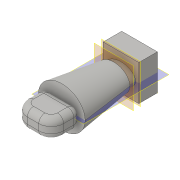
# Autodesk Inventor part: maleNT2
Saved by Autodesk Inventor 2016 (Build 200138000, 138)
## iProperties
Created: 2016-01-27
Part Number: maleNT2
Material: Generic
Document SubType Name: Modeling
Designer: 301278
Density: 1 g/cm^3
Appearance: Default
Author: 301278
Autodesk Inventor part; units mm, degrees
ref_plane "YZ Plane" through (0, 0, 0) normal (1, 0, 0) x (0, 1, 0)
ref_plane "XZ Plane" through (0, 0, 0) normal (0, 1, 0) x (-1, 0, 0)
ref_plane "XY Plane" through (0, 0, 0) normal (0, 0, 1) x (1, 0, 0)
sketch "Sketch1" plane through (0, 0, 0) normal (0, 0, 1) x (1, 0, 0)
  line L0 (0, 0) -> (14.605, 0)
  line L1 (14.605, 0) -> (14.605, 14.605)
  line L2 (14.605, 14.605) -> (0, 14.605)
  line L3 (0, 14.605) -> (0, 0)
  dimension "d0" = 14.605
  dimension "d1" = 14.605
  constraints: 8 end point, 2 parallel, 1 horizontal, 1 perpendicular
  measures "d0" distance of L2.end L1.end
  measures "d1" distance of L1.end L0.end
extrude "Extrusion1" add sketch "Sketch1" along normal blind 7.62
ref_plane "Work Plane1" through (0, 14.605, 7.62) normal (0, 0, 1) x (1, 0, 0)
sketch "Sketch2" plane through (0, 14.605, 7.62) normal (0, 0, 1) x (1, 0, 0)
  line L0 (14.605, 0) -> (0, 0) construction
  line L1 (0, 0) -> (7.3025, 0) construction
  line L2 (7.3025, 0) -> (14.605, 0) construction
  line L3 (7.3025, 0) -> (7.3025, -7.3025) construction
  ellipse E0 centre (7.3025, -7.3025) end of major axis (13.2969, -7.3025) minor radius 3.937
  point P0 (0, -14.605)
  dimension "d7" = 5.9944
  dimension "d8" = 3.937
  dimension "d4" = 7.3025
  dimension "d5" = 7.3025
  dimension "d6" = 7.3025
  constraints: 6 end point, 1 coincident, 1 collinear, 1 midpoint, 1 perpendicular, 2 other
  measures "d4" distance of L0.end L1.end
  measures "d5" distance of L1.end L0.start
  measures "d6" distance of L1.end L3.end
extrude "Extrusion2" add sketch "Sketch2" along normal blind 2.921
ref_plane "Work Plane2" through (0, 14.605, 10.541) normal (0, 0, 1) x (1, 0, 0)
sketch "Sketch3" plane through (0, 14.605, 10.541) normal (0, 0, 1) x (1, 0, 0)
  ellipse E0 centre (7.3025, -7.3076) end of major axis (13.8567, -7.3076) minor radius 5.2829
  ellipse E1 centre (7.3025, -7.3025) end of major axis (1.3081, -7.3025) minor radius 3.937 projected
  point P0 (0, -14.605)
  dimension "d12" = 0
  constraints: 3 other
  measures "d12" horizontal distance of point (7.302, -7.302) point (7.302, -7.308)
extrude "Extrusion3" add sketch "Sketch3" along normal blind 21.336 draft 8 contours E0 | E1
sketch "Sketch4" plane through (0, 0, 0) normal (0, -1, 0) x (1, 0, 0)
  point P0 (0, 0)
sketch "Sketch5" plane through (0, 0, 0) normal (0, -1, 0) x (1, 0, 0)
  line L0 (14.605, 0) -> (0, 0) projected
ref_plane "Work Plane3" through (7.3025, 7.3025, 10.541) normal (0, -1, 0) x (0, 0, 1)
sketch "Sketch6" plane through (7.3025, 7.3025, 10.541) normal (0, -1, 0) x (0, 0, 1)
  point P0 (-10.541, 7.3025)
sketch "Sketch7" plane through (7.3025, 7.3025, 10.541) normal (0, -1, 0) x (0, 0, 1)
  point P0 (-10.541, 7.3025)
sketch "Sketch8" plane through (7.3025, 7.3025, 10.541) normal (0, -1, 0) x (0, 0, 1)
  line L0 (21.4205, -0.1285) -> (33.2425, -0.1285)
  line L1 (33.2425, -0.1285) -> (33.2425, 7.3025)
  line L2 (33.2425, 7.3025) -> (21.4205, 7.3025)
  line L3 (21.4205, 7.3025) -> (21.4205, -0.1285)
  line L4 (33.2425, -0.1285) -> (33.2425, -7.5594)
  line L5 (33.2425, -7.5594) -> (21.4205, -7.5594)
  line L6 (21.4205, -7.5594) -> (21.4205, -0.1285)
  point P0 (-10.541, 7.3025)
  constraints: 14 end point, 2 parallel, 2 symmetric about line, 1 horizontal, 1 perpendicular
extrude "Extrusion4" add sketch "Sketch8" along normal mid plane 7.62
fillet "Fillet1" radius 5.08 1 edges at (0, 7.3025, 43.7835)
fillet "Fillet2" radius 5.08 1 edges at (14.8619, 7.3025, 43.7835)
fillet "Fillet3" radius 2.54 5 edges at (7.431, 3.4925, 43.7835) (1.4879, 3.4925, 42.2956) (0, 3.4925, 35.3325) (13.374, 3.4925, 42.2956) (14.8619, 3.4925, 35.3325)
fillet "Fillet4" radius 2.54 5 edges at (7.431, 11.1125, 43.7835) (13.374, 11.1125, 42.2956) (14.8619, 11.1125, 35.3325) (1.4879, 11.1125, 42.2956) (0, 11.1125, 35.3325)
fillet "Fillet5" radius 2.54 6 edges at (7.431, 11.1125, 31.9615) (0.7439, 10.3686, 31.9615) (0, 7.3025, 31.9615) (0.7439, 4.2364, 31.9615) (7.431, 3.4925, 31.9615) (14.8619, 7.3025, 31.9615)
body "Solid1"
